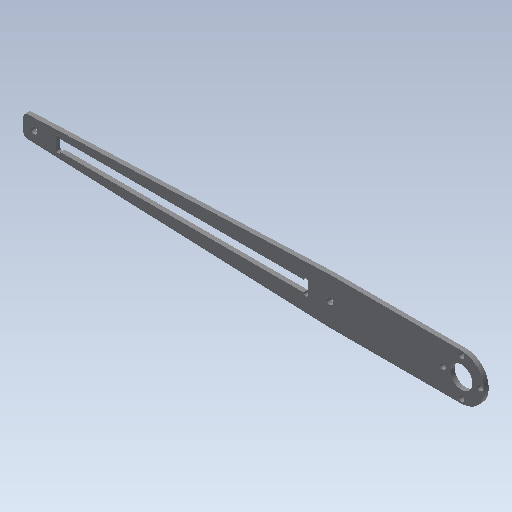
# Autodesk Inventor part: 前腕_メインフレーム_1_1
Saved by Autodesk Inventor 2020.3 (Build 243373000, 373)
## iProperties
Created: 2016-05-04
Part Number: 前腕_メインフレーム_1_1
Material: GFRP
Document SubType Name: Modeling
Designer: hiroaki
Density: 1.75 g/cm^3
Appearance: 滑らか - 淡い灰色
Mass: 10.0158 g
Surface Area: 72.6648 cm^2
Volume: 5.7233 cm^3
Category: 前腕
d0: 200.000 mm
d1: 3.100 mm
d2: 21.000 mm
d3: 10.000 mm
d4: 5.000 mm
d5: 12.000 mm
d6: 135.000 mm
d7: 5.000 mm
d8: 0.050 mm
d9: 2.100 mm
d10: 2.700 mm
d11: 8.500 mm
d12: 10.100 mm
d13: 4.000 ul
d15: 360.00 deg
d17: 2.000 mm
d18: 0.00 deg
d19: 2.000 mm
Author: hiroaki
Autodesk Inventor part; units mm, degrees
ref_plane "YZ Plane" through (0, 0, 0) normal (1, 0, 0) x (0, 1, 0)
ref_plane "XZ Plane" through (0, 0, 0) normal (0, 1, 0) x (-1, 0, 0)
ref_plane "XY Plane" through (0, 0, 0) normal (0, 0, 1) x (1, 0, 0)
sketch "スケッチ1" plane through (0, 0, 0) normal (0, 0, 1) x (1, 0, 0)
  circle A0 centre (0, 0) radius 10.5 construction
  line L0 (0, 10.5) -> (-200, 10.5) construction
  line L1 (-200, 10.5) -> (-200, -10.5) construction
  line L2 (-200, -10.5) -> (0, -10.5) construction
  circle A1 centre (-195, 0) radius 1.55
  line L3 (-185, 2.5) -> (-70, 2.5) construction
  line L4 (-70, 2.5) -> (-70, -2.5) construction
  line L5 (-70, -2.5) -> (-185, -2.5) construction
  line L6 (-185, -2.5) -> (-185, 2.5) construction
  line L7 (-127.5, 2.5) -> (-127.5, -2.5) construction
  circle A2 centre (-60, 0) radius 1.55
  line L8 (-12, 21.3027) -> (-12, -27.3903) construction
  line L9 (-69.95, 2.55) -> (-185.05, 2.55) construction
  line L10 (-185.05, 2.55) -> (-185.05, -2.55) construction
  line L11 (-185.05, -2.55) -> (-69.95, -2.55) construction
  line L12 (-69.95, -2.55) -> (-69.95, 2.55) construction
  circle A3 centre (-184, 2.55) radius 1.05 construction
  line L13 (-185, 0) -> (-127.5, 0) construction
  line L14 (-185.05, 2.55) -> (-185.05, -2.55)
  arc A4 (-182.95, 2.55) -> (-185.05, 2.55) centre (-184, 2.55) ccw
  line L15 (-182.95, 2.55) -> (-72.05, 2.55)
  arc A5 (-69.95, 2.55) -> (-72.05, 2.55) centre (-71, 2.55) ccw
  line L16 (-69.95, 2.55) -> (-69.95, -2.55)
  arc A6 (-185.05, -2.55) -> (-182.95, -2.55) centre (-184, -2.55) ccw
  line L17 (-182.95, -2.55) -> (-72.05, -2.55)
  arc A7 (-72.05, -2.55) -> (-69.95, -2.55) centre (-71, -2.55) ccw
  circle A8 centre (0, 8.5) radius 1.35
  circle A9 centre (0, 0) radius 5.05
  circle A10 centre (-8.5, 0) radius 1.35
  circle A11 centre (0, -8.5) radius 1.35
  circle A12 centre (8.5, 0) radius 1.35
  line L18 (-200, 4.8006) -> (-200, -4.8006)
  line L19 (-200, 4.8006) -> (-60, 10.5)
  line L20 (-60, 10.5) -> (0, 10.5)
  line L21 (-200, -4.8006) -> (-60, -10.5)
  line L22 (-60, -10.5) -> (0, -10.5)
  arc A13 (0, -10.5) -> (0, 10.5) centre (0, 0) ccw
  circle A14 centre (-195, 0) radius 5 construction
  point P0 (-200, 0)
  dimension "d9" = 2.1
  dimension "d0" = 200
  dimension "d1" = 3.1
  dimension "d2" = 21
  dimension "d3" = 10
  dimension "d4" = 5
  dimension "d5" = 12
  dimension "d6" = 135
  dimension "d7" = 5
  dimension "d8" = 0.05
  dimension "d10" = 2.7
  dimension "d11" = 8.5
  dimension "d12" = 10.1
  dimension "d15" = 360
  constraints: 46 end point, 13 centre point, 12 point on circle, 7 tangent, 6 midpoint, 5 coincident, 5 horizontal, 5 symmetric about line, 4 horizontal alignment, 4 parallel, 4 perpendicular, 4 vertical, 3 equal radius, 2 collinear, 2 vertical alignment, 1 concentric, 1 point on line, 19 other
  measures "d0" distance from line of L1 point (0, 0)
  measures "d1" diameter of A1
  measures "d2" distance of L0.end L1.end
  measures "d3" distance from line of L6 A1.centre
  measures "d4" distance from line of L1 A1.centre
  measures "d5" distance from line of point (0, 0) L8
  measures "d6" distance of A2.centre A1.centre
  measures "d7" distance of L3.end L4.end
  measures "d8" distance between parallel lines of L9 L3
  measures "d10" diameter of A8
  measures "d11" distance of point (0, 0) A8.centre
  measures "d12" diameter of A9
extrude "押し出し1" add sketch "スケッチ1" along normal blind 2
fillet "フィレット1" radius 2 2 edges at (-200, -4.8006, 1) (-200, 4.8006, 1)
equation "\"H_head\" = 28.5"
equation "\"H_leg\" = 199.5"
equation "\"足の面積\" = 12720.125"
equation "\"現在の面積\" = 11560"
equation "\"足_短辺\" = 68"
equation "\"円柱\" = 313.5"
equation "\"胴体中心から手先\" = 342"
equation "\"H_leg_1\" = 186.2"
equation "\"H_leg_MAX\" = 399"
equation "\"H_head_1\" = 26.6"
equation "\"H_head_MAX\" = 142.5"
